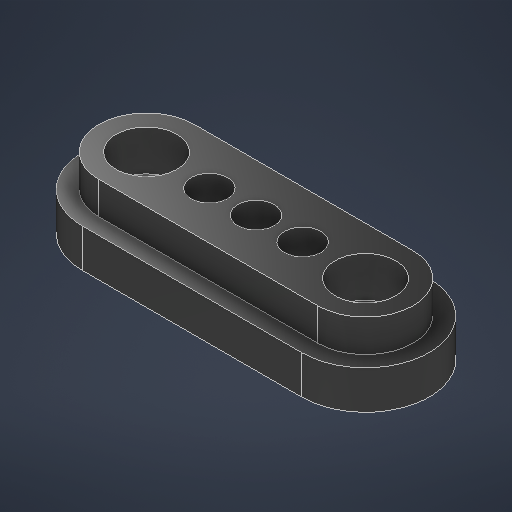
# Autodesk Inventor part: Pogo1
Saved by Autodesk Inventor 2026 (Build 300175000, 175)
## iProperties
Created: 2025-04-17
Part Number: Pogo1
Material: Nylon 6
Document SubType Name: Modeling
Designer: ct_vi
Density: 1.12 g/cm^3
Appearance: Nylon 6
Author: ct_vi
Autodesk Inventor part; units mm, degrees
ref_plane "YZ Plane" through (0, 0, 0) normal (1, 0, 0) x (0, 1, 0)
ref_plane "XZ Plane" through (0, 0, 0) normal (0, 1, 0) x (-1, 0, 0)
ref_plane "XY Plane" through (0, 0, 0) normal (0, 0, 1) x (1, 0, 0)
sketch "Sketch2" plane through (0, 0, 0) normal (0, 1, 0) x (-1, 0, 0)
  line L0 (-13.1182, 6.5103) -> (18.7692, 6.5103) construction
  line L1 (18.7692, 6.5103) -> (18.7692, -12.5367) construction
  line L2 (18.7692, -12.5367) -> (-13.1182, -12.5367) construction
  line L3 (-13.1182, -12.5367) -> (-13.1182, 6.5103) construction
  line L4 (-5.4, 3.15) -> (5.4, 3.15)
  line L5 (8.55, 0) -> (8.55, 0)
  line L6 (5.4, -3.15) -> (-5.4, -3.15)
  line L7 (-8.55, 0) -> (-8.55, 0)
  line L8 (-8.55, 3.15) -> (8.55, -3.15) construction
  line L9 (8.55, 3.15) -> (-8.55, -3.15) construction
  arc A0 (8.55, 0) -> (5.4, 3.15) centre (5.4, 0) ccw
  arc A1 (5.4, -3.15) -> (8.55, 0) centre (5.4, 0) ccw
  arc A2 (-5.4, 3.15) -> (-8.55, 0) centre (-5.4, 0) ccw
  arc A3 (-8.55, 0) -> (-5.4, -3.15) centre (-5.4, 0) ccw
  line L10 (5.4, 2.35) -> (-5.4, 2.35)
  line L11 (-7.75, 0) -> (-7.75, 0)
  line L12 (-5.4, -2.35) -> (5.4, -2.35)
  line L13 (7.75, 0) -> (7.75, 0)
  line L14 (7.75, 2.35) -> (-7.75, -2.35) construction
  line L15 (-7.75, 2.35) -> (7.75, -2.35) construction
  arc A4 (-5.4, 2.35) -> (-7.75, 0) centre (-5.4, 0) ccw
  arc A5 (-7.75, 0) -> (-5.4, -2.35) centre (-5.4, 0) ccw
  arc A6 (7.75, 0) -> (5.4, 2.35) centre (5.4, 0) ccw
  arc A7 (5.4, -2.35) -> (7.75, 0) centre (5.4, 0) ccw
  circle A8 centre (5.4, 0) radius 1.5
  circle A9 centre (-5.4, 0) radius 1.5
  circle A10 centre (2.3, 0) radius 0.9
  circle A11 centre (0, 0) radius 0.9
  circle A12 centre (-2.3, 0) radius 0.9
  circle A13 centre (2.3, 0) radius 0.35
  circle A14 centre (0, 0) radius 0.35
  circle A15 centre (-2.3, 0) radius 0.35
  point P0 (-7.75, 0)
  point P1 (7.75, 0)
  point P2 (-8.55, 0)
  point P3 (8.55, 0)
  dimension "d61" = 17.1
  dimension "d62" = 6.3
  dimension "d88" = 3.15
  dimension "d90" = 0.8
  dimension "d91" = 0.8
  dimension "d92" = 2.35
  dimension "d93" = 3
  dimension "d94" = 3
  dimension "d97" = 1.8
  dimension "d98" = 1.8
  dimension "d99" = 1.8
  dimension "d100" = 4.6
  dimension "d115" = 0.7
  dimension "d116" = 0.7
  dimension "d117" = 0.7
  constraints: 24 end point, 16 centre point, 16 point on circle, 16 point on line, 16 tangent, 6 coincident, 6 equal radius, 4 midpoint, 4 parallel, 2 horizontal, 2 perpendicular, 2 other
  measures "d61" distance of L8.end L9.end
  measures "d62" distance of L9.start L8.end
  measures "d88" radius of A0
  measures "d90" distance between parallel lines of L4 L10
  measures "d91" distance from line of L7.end L11
  measures "d92" radius of A4
  measures "d93" diameter of A8
  measures "d94" diameter of A9
  measures "d97" diameter of A10
  measures "d98" diameter of A11
  measures "d99" diameter of A12
  measures "d100" distance of A12.centre A10.centre
  measures "d115" diameter of A13
  measures "d116" diameter of A14
  measures "d117" diameter of A15
extrude "Extrusion1" add sketch "Sketch2" along normal blind 3.5 contours A6 A7 L12 A5 A4 L10 | A8 | A9 | A10 | A11 | A12 | A13 | A14 | A15
extrude "Extrusion2" add sketch "Sketch2" along normal blind 1.9 contours L4 A0 A1 L6 A3 A2
extrude "Extrusion3" cut sketch "Sketch2" along normal through all contours A10 | A11 | A12 | A13 | A14 | A15
ref_plane "Work Plane1" through (0, -1.5, 0) normal (0, -1, 0) x (1, 0, 0)
extrude "Extrusion5" add sketch "Sketch2" along normal blind 2 contours A10 | A11 | A12
sketch "Sketch5" plane through (0, 3.5, 0) normal (0, 1, 0) x (1, 0, 0)
  line L0 (0, 0) -> (5.4, 0)
  circle A0 centre (5.4, 0) radius 1.5
  line L1 (0, 0) -> (-5.4, 0)
  circle A1 centre (-5.4, 0) radius 1.5
  dimension "d127" = 5.4
  dimension "d128" = 3
  dimension "d129" = 5.4
  dimension "d130" = 3
  constraints: 4 end point, 2 centre point, 2 coincident, 2 horizontal
  measures "d127" distance of L0.start L0.end
  measures "d128" diameter of A0
  measures "d129" distance of L0.start L1.end
  measures "d130" diameter of A1
extrude "Extrusion7" cut sketch "Sketch5" against normal blind 2
body "Solid1"
